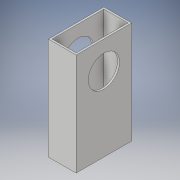
# Autodesk Inventor part: anchor point
Saved by Autodesk Inventor 2018 (Build 220112000, 112)
## iProperties
Created: 2020-01-25
Part Number: anchor point
Material: Generic
Document SubType Name: Modeling
Designer: s-2513225
Density: 1 g/cm^3
Appearance: Default
Author: s-2513225
Autodesk Inventor part; units mm, degrees
ref_plane "YZ Plane" through (0, 0, 0) normal (1, 0, 0) x (0, 1, 0)
ref_plane "XZ Plane" through (0, 0, 0) normal (0, 1, 0) x (-1, 0, 0)
ref_plane "XY Plane" through (0, 0, 0) normal (0, 0, 1) x (1, 0, 0)
sketch "Sketch2" plane through (0, 0, 0) normal (0, 1, 0) x (-1, 0, 0)
  line L0 (0, 0) -> (-25.4, 0)
  line L1 (-25.4, 0) -> (-25.4, -50.8)
  line L2 (-25.4, -50.8) -> (0, -50.8)
  line L3 (0, -50.8) -> (0, 0)
  line L4 (-1.778, -1.778) -> (-23.622, -1.778)
  line L5 (-23.622, -1.778) -> (-23.622, -49.022)
  line L6 (-23.622, -49.022) -> (-1.778, -49.022)
  line L7 (-1.778, -49.022) -> (-1.778, -1.778)
  dimension "d0" = 25.4
  dimension "d1" = 50.8
  dimension "d2" = 1.778
  constraints: 16 end point, 4 parallel, 2 perpendicular, 1 horizontal, 3 other
  measures "d0" distance of L2.end L1.end
  measures "d1" distance of L1.end L0.end
  measures "d2" distance between parallel lines of L3 L7
extrude "Extrusion1" add sketch "Sketch2" along normal blind 93.345
sketch "Sketch3" plane through (25.4, 0, 0) normal (1, 0, 0) x (0, 0, -1)
  line L0 (1.778, 0) -> (49.022, 0) construction
  line L1 (25.4, 0) -> (25.4, 42.545) construction
  line L2 (25.4, 42.545) -> (25.4, 67.945) construction
  circle A0 centre (25.4, 67.945) radius 14.2875
  point P0 (0, 0)
  dimension "d5" = 42.545
  dimension "d6" = 25.4
  dimension "d7" = 28.575
  constraints: 4 end point, 2 vertical, 1 centre point, 1 coincident, 1 midpoint
  measures "d5" distance of L1.start L1.end
  measures "d6" distance of L1.end L2.end
  measures "d7" diameter of A0
extrude "Extrusion2" cut sketch "Sketch3" against normal blind 42.545
body "Solid1"
